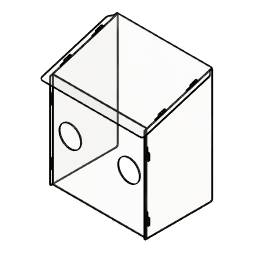
Polycarbinate Box - Flatpack - V5 v38 (Autodesk Fusion 360 design; units mm, degrees)
Autodesk Fusion 360 part; units mm, degrees
note: some values were not read from the file. Set by a fixed rule: which sketch regions a step uses.
ref_plane "WorkPlane1" through (474.6, 0, 0) normal (1, 0, 0) x (0, 1, 0)
ref_plane "WorkPlane2" through (0, 0, 500) normal (0, 0, 1) x (1, 0, 0)
ref_plane "WorkPlane3" through (0, 0, 0) normal (1, 0, 0) x (0, 1, 0)
ref_plane "WorkPlane4" through (0, 400, 0) normal (0, 1, 0) x (0, 0, 1)
sketch "Sketch1" plane through (0, 0, 0) normal (1, 0, 0) x (0, 1, 0)
  line L0 (0, 483.1819) -> (0, 0)
  line L1 (0, 0) -> (390.6577, 0)
  line L2 (9.525, 393.7) -> (14.2875, 393.7)
  line L3 (14.2875, 393.7) -> (14.2875, 355.6)
  line L4 (14.2875, 355.6) -> (9.525, 355.6)
  line L5 (9.525, 355.6) -> (9.525, 393.7)
  line L6 (9.525, 114.3) -> (14.2875, 114.3)
  line L7 (14.2875, 114.3) -> (14.2875, 76.2)
  line L8 (14.2875, 76.2) -> (9.525, 76.2)
  line L9 (9.525, 76.2) -> (9.525, 114.3)
  arc A0 (390.6577, 0) -> (400.1827, 9.525) centre (390.6577, 9.525) ccw
  line L10 (0, 483.1819) -> (336.55, 586.2176)
  line L11 (72.8618, 492.2069) -> (69.144, 504.3505)
  line L12 (104.8626, 506.9847) -> (102.539, 514.5745)
  line L13 (89.5593, 497.3188) -> (88.1651, 501.8727)
  line L14 (104.8626, 506.9847) -> (88.1651, 501.8727)
  line L15 (230.2932, 540.4049) -> (226.5754, 552.5485)
  line L16 (246.9907, 545.5169) -> (245.5965, 550.0707)
  line L17 (245.5965, 550.0707) -> (262.294, 555.1827)
  line L18 (262.294, 555.1827) -> (259.9704, 562.7725)
  line L19 (72.8618, 492.2069) -> (0, 469.9)
  line L20 (336.55, 572.9357) -> (246.9907, 545.5169)
  line L21 (230.2932, 540.4049) -> (89.5593, 497.3188)
  line L22 (336.55, -28.3525) -> (336.55, 572.9357)
  line L23 (89.5593, 497.3188) -> (88.1651, 501.8727)
  dimension "d6" = 9.525
  dimension "d7" = 76.2
  dimension "d8" = 38.1
  dimension "d9" = 4.7625
  dimension "d13" = 9.525
  dimension "d14" = 4.7625
  dimension "d15" = 38.1
  dimension "d31" = 9.525
  dimension "d140" = 76.2
  dimension "d150" = 469.9
  dimension "d151" = 12.7
  dimension "d152" = 76.2
  dimension "d153" = 34.925
  dimension "d154" = 17.4625
  dimension "d155" = 4.7625
  dimension "d160" = 34.925
  dimension "d161" = 17.4625
  dimension "d163" = 4.7625
  dimension "d165" = 76.2
  dimension "d202" = 336.55
  constraint vertical L0
  constraint horizontal L1
  constraint coincident L0.end L1.start
  constraint coincident L0 L19.end
  constraint horizontal L2
  constraint vertical L3
  constraint horizontal L4
  constraint vertical L5
  constraint horizontal L6
  constraint vertical L7
  constraint horizontal L8
  constraint vertical L9
  constraint tangent L1 A0
  constraint perpendicular L1 L22
  constraint coincident L11.start L20
  constraint coincident L10 L11.end
  constraint perpendicular L10 L11
  constraint coincident L10 L12.end
  constraint perpendicular L10 L12
  constraint perpendicular L13 L14
  constraint coincident L10.end L22
  constraint coincident L15.start L20
  constraint coincident L10 L15.end
  constraint perpendicular L10 L15
  constraint perpendicular L16 L20
  constraint perpendicular L16 L17
  constraint coincident L10 L18.end
  constraint perpendicular L10 L18
  constraint collinear L19 L20
  constraint collinear L20 L21
  measures "d6" distance of L0 L9
  measures "d7" distance of L1 L8
  measures "d8" distance of L6.start L8.end
  measures "d9" distance of L7 L9
  measures "d13" distance of L0 L5
  measures "d14" distance of L3 L5
  measures "d15" distance of L2.start L4.end
  measures "d31" radius of A0
  measures "d140" distance of L19.end L2
  measures "d150" distance of L1 L19.end
  measures "d151" distance of L10 L20
  measures "d152" distance of L19.end L11
  measures "d153" distance of L11 L12
  measures "d154" distance of L11 L13
  measures "d155" distance of L14 L20
  measures "d160" distance of L15 L18
  measures "d161" distance of L15 L16
  measures "d163" distance of L17 L20
  measures "d165" distance of L20.start L18
  measures "d202" distance of L0 L22
extrude "Extrude1" add sketch "Sketch1" along normal blind 4.7625 contours L0 L1 L10 L11 L12 L13 L14 L15 L16 L17 L18 L19 L20 L21 L22 L23 makes body 1
fillet "Fillet1" radius 3.175 6 edges at (2.3813, 69.144, 504.3505) (2.3813, 102.539, 514.5745) (2.3813, 104.8626, 506.9847) (2.3813, 226.5754, 552.5485) (2.3813, 259.9704, 562.7725) (2.3813, 262.294, 555.1827) on bodies 1
fillet "Fillet2" radius 1.5875 5 edges at (2.3813, 0, 469.9) (2.3813, 336.55, 572.9357) (2.3813, 0, 0) (2.3813, 72.8618, 492.2069) (2.3813, 230.2932, 540.4049) on bodies 1
fillet "Fillet3" radius 9.525 1 edges at (2.3813, 336.55, 0) on bodies 1
sketch "Sketch2" plane through (4.7625, 0, 0) normal (1, 0, 0) x (0, 1, 0)
  line L0 (1.5875, 0) -> (327.025, 0)
  arc A0 (14.2875, 114.3) -> (11.1125, 114.3) centre (12.7, 114.3) ccw
  line L1 (9.525, 114.3) -> (14.2875, 114.3)
  arc A1 (9.525, 114.3) -> (9.525, 111.125) centre (9.525, 112.7125) ccw
  arc A2 (9.525, 79.375) -> (9.525, 76.2) centre (9.525, 77.7875) ccw
  arc A3 (11.1125, 76.2) -> (14.2875, 76.2) centre (12.7, 76.2) ccw
  arc A4 (9.525, 358.775) -> (9.525, 355.6) centre (9.525, 357.1875) ccw
  line L2 (14.2875, 355.6) -> (9.525, 355.6)
  line L3 (9.525, 355.6) -> (9.525, 393.7)
  line L4 (9.525, 393.7) -> (14.2875, 393.7)
  arc A5 (11.1125, 355.6) -> (14.2875, 355.6) centre (12.7, 355.6) ccw
  arc A6 (14.2875, 393.7) -> (11.1125, 393.7) centre (12.7, 393.7) ccw
  arc A7 (9.525, 393.7) -> (9.525, 390.525) centre (9.525, 392.1125) ccw
  line L5 (14.2875, 393.7) -> (14.2875, 355.6)
  line L6 (336.55, 9.525) -> (336.55, 570.7895)
  arc A8 (327.025, 0) -> (336.55, 9.525) centre (327.025, 9.525) ccw
  arc A9 (336.55, 570.7895) -> (334.4978, 572.3074) centre (334.9625, 570.7895) ccw
  line L7 (334.4978, 572.3074) -> (246.9907, 545.5169)
  line L8 (246.9907, 545.5169) -> (245.5965, 550.0707)
  line L9 (245.5965, 550.0707) -> (259.2581, 554.2533)
  arc A10 (259.2581, 554.2533) -> (261.3645, 558.2186) centre (258.3286, 557.2892) ccw
  line L10 (261.3645, 558.2186) -> (260.8998, 559.7366)
  arc A11 (260.8998, 559.7366) -> (256.9345, 561.843) centre (257.8639, 558.8071) ccw
  line L11 (256.9345, 561.843) -> (229.6113, 553.478)
  arc A12 (229.6113, 553.478) -> (227.5048, 549.5126) centre (230.5407, 550.4421) ccw
  line L12 (227.5048, 549.5126) -> (229.8285, 541.9229)
  arc A13 (228.7752, 539.9402) -> (229.8285, 541.9229) centre (228.3105, 541.4581) ccw
  line L13 (228.7752, 539.9402) -> (89.5593, 497.3188)
  line L14 (89.5593, 497.3188) -> (88.1651, 501.8727)
  line L15 (88.1651, 501.8727) -> (101.8267, 506.0552)
  arc A14 (101.8267, 506.0552) -> (103.9332, 510.0206) centre (100.8973, 509.0911) ccw
  line L16 (103.9332, 510.0206) -> (103.4685, 511.5386)
  arc A15 (103.4685, 511.5386) -> (99.5031, 513.645) centre (100.4326, 510.6091) ccw
  line L17 (99.5031, 513.645) -> (72.1799, 505.2799)
  arc A16 (72.1799, 505.2799) -> (70.0735, 501.3146) centre (73.1094, 502.244) ccw
  line L18 (70.0735, 501.3146) -> (72.3971, 493.7248)
  arc A17 (71.3439, 491.7421) -> (72.3971, 493.7248) centre (70.8791, 493.2601) ccw
  line L19 (71.3439, 491.7421) -> (1.1228, 470.2437)
  arc A18 (1.1228, 470.2437) -> (0, 468.7258) centre (1.5875, 468.7258) ccw
  line L20 (0, 468.7258) -> (0, 1.5875)
  arc A19 (0, 1.5875) -> (1.5875, 0) centre (1.5875, 1.5875) ccw
  arc A20 (248.6324, 551.0002) -> (245.5965, 550.0707) centre (247.1145, 550.5355) ccw
  line L21 (246.0605, 548.5552) -> (242.3336, 547.4142)
  line L22 (246.9899, 545.5193) -> (245.5965, 550.0707)
  arc A21 (246.0605, 548.5552) -> (246.9899, 545.5193) centre (246.5252, 547.0372) ccw
  line L23 (248.6324, 551.0002) -> (247.4641, 554.8162)
  line L24 (14.2875, 355.6) -> (9.525, 355.6)
  line L25 (9.525, 355.6) -> (9.525, 393.7)
  line L26 (9.525, 393.7) -> (14.2875, 393.7)
  line L27 (14.2875, 393.7) -> (14.2875, 355.6)
  line L28 (14.2875, 76.2) -> (9.525, 76.2)
  line L29 (9.525, 76.2) -> (9.525, 114.3)
  line L30 (9.525, 114.3) -> (14.2875, 114.3)
  line L31 (14.2875, 114.3) -> (14.2875, 76.2)
  line L32 (91.201, 502.8022) -> (90.0328, 506.6182)
  arc A22 (88.6291, 500.3571) -> (89.5586, 497.3212) centre (89.0939, 498.8392) ccw
  arc A23 (91.201, 502.8022) -> (88.1651, 501.8727) centre (89.6831, 502.3374) ccw
  line L33 (88.6291, 500.3571) -> (84.9022, 499.2161)
  dimension "d173" = 3.175
  constraint coincident L21.start L22
  constraint perpendicular L21 L22
  constraint tangent A20 L23
  constraint tangent A20 L22
  constraint tangent L21 A21
  constraint coincident L22.start A21.end
  constraint tangent L32 A23
  constraint tangent A22 L33
  measures "d173" distance of L22 L23
extrude "Extrude2" cut sketch "Sketch2" against normal blind 7.62 contours L8 L22 A21 | L9 A20 | L15 A23 | L14 A22 | A0 L1 L30 | A3 L28 | A1 L29 | A2 L29 | A4 L3 L25 | L3 A7 L25 | L2 A5 L24 | L4 A6 L26 bodies 1
ref_plane "WorkPlane5" through (237.3, 168.275, 286.4678) normal (-1, 0, 0) x (0, -1, 0)
mirror "Mirror1" about plane through (237.3, 168.275, 286.4678) normal (-1, 0, 0) of bodies 1 makes body 2
sketch "Sketch3" plane through (0, 14.2875, 0) normal (0, -1, 0) x (1, 0, 0)
  line L0 (495.2375, 0) -> (4.7625, 0)
  line L1 (4.7625, 474.2742) -> (469.8375, 474.2742)
  line L2 (237.3, 644.4156) -> (237.3, -18.4393)
  line L3 (4.7625, 76.2) -> (4.7625, 0)
  line L4 (4.7625, 1.5875) -> (4.7625, 0)
  line L5 (4.7625, 9.525) -> (4.7625, 0)
  line L6 (4.7625, 93.6625) -> (-9.525, 93.6625)
  line L7 (-9.525, 93.6625) -> (-9.525, 58.7375)
  line L8 (-9.525, 58.7375) -> (0, 58.7375)
  line L9 (0, 58.7375) -> (0, 76.2)
  line L10 (0, 76.2) -> (4.7625, 76.2)
  line L11 (0, 393.7) -> (0, 355.6)
  line L12 (0, 355.6) -> (4.7625, 355.6)
  line L13 (4.7625, 355.6) -> (4.7625, 393.7)
  line L14 (4.7625, 393.7) -> (0, 393.7)
  line L15 (-9.525, 373.0625) -> (-9.525, 338.1375)
  line L16 (0, 355.6) -> (4.7625, 355.6)
  line L17 (4.7625, 373.0625) -> (0, 373.0625)
  line L18 (4.7625, 373.0625) -> (-9.525, 373.0625)
  line L19 (0, 338.1375) -> (0, 355.6)
  line L20 (-9.525, 338.1375) -> (0, 338.1375)
  line L21 (4.7625, 373.0625) -> (4.7625, 474.2742)
  line L22 (4.7625, 355.6) -> (4.7625, 93.6625)
  line L23 (0, 114.3) -> (0, 76.2)
  line L24 (0, 76.2) -> (4.7625, 76.2)
  line L25 (4.7625, 76.2) -> (4.7625, 114.3)
  line L26 (4.7625, 114.3) -> (0, 114.3)
  line L27 (237.3, 474.2742) -> (237.3, 298.45)
  line L28 (4.7625, 474.2742) -> (0, 474.2742)
  line L29 (4.7625, 500.3571) -> (4.7625, 501.8727)
  line L30 (469.8375, 497.3212) -> (469.8375, 497.3188)
  line L31 (469.8375, 545.5193) -> (469.8375, 545.5169)
  line L32 (474.6, 393.7) -> (474.6, 355.6)
  line L33 (474.6, 76.2) -> (469.8375, 76.2)
  line L34 (474.6, 355.6) -> (469.8375, 355.6)
  line L35 (474.6, 114.3) -> (474.6, 76.2)
  line L36 (474.6, 355.6) -> (469.8375, 355.6)
  line L37 (474.6, 338.1375) -> (474.6, 355.6)
  line L38 (469.8375, 373.0625) -> (469.8375, 474.2742)
  line L39 (469.8375, 474.2742) -> (474.6, 474.2742)
  line L40 (484.125, 373.0625) -> (484.125, 338.1375)
  line L41 (469.8375, 76.2) -> (469.8375, 114.3)
  line L42 (469.8375, 355.6) -> (469.8375, 93.6625)
  line L43 (484.125, 338.1375) -> (474.6, 338.1375)
  line L44 (469.8375, 373.0625) -> (474.6, 373.0625)
  line L45 (469.8375, 76.2) -> (469.8375, 0)
  line L46 (484.125, 58.7375) -> (474.6, 58.7375)
  line L47 (469.8375, 373.0625) -> (484.125, 373.0625)
  line L48 (469.8375, 1.5875) -> (469.8375, 0)
  line L49 (469.8375, 393.7) -> (474.6, 393.7)
  line L50 (474.6, 58.7375) -> (474.6, 76.2)
  line L51 (469.8375, 500.3571) -> (469.8375, 501.8727)
  line L52 (469.8375, 93.6625) -> (484.125, 93.6625)
  line L53 (484.125, 93.6625) -> (484.125, 58.7375)
  line L54 (469.8375, 114.3) -> (474.6, 114.3)
  line L55 (469.8375, 9.525) -> (469.8375, 0)
  line L56 (474.6, 76.2) -> (469.8375, 76.2)
  line L57 (469.8375, 355.6) -> (469.8375, 393.7)
  line L58 (4.7625, 548.5552) -> (4.7625, 550.0707)
  arc A0 (4.7625, 355.6) -> (1.5875, 355.6) centre (3.175, 355.6) ccw
  arc A1 (0, 355.6) -> (0, 352.425) centre (0, 354.0125) ccw
  arc A2 (4.7625, 76.2) -> (1.5875, 76.2) centre (3.175, 76.2) ccw
  arc A3 (0, 76.2) -> (0, 73.025) centre (0, 74.6125) ccw
  arc A4 (473.0125, 76.2) -> (469.8375, 76.2) centre (471.425, 76.2) ccw
  arc A5 (474.6, 73.025) -> (474.6, 76.2) centre (474.6, 74.6125) ccw
  arc A6 (473.0125, 355.6) -> (469.8375, 355.6) centre (471.425, 355.6) ccw
  arc A7 (474.6, 352.425) -> (474.6, 355.6) centre (474.6, 354.0125) ccw
  point P0 (4.7625, 393.7)
  point P1 (4.7625, 355.6)
  point P2 (4.7625, 114.3)
  point P3 (4.7625, 76.2)
  point P4 (469.8375, 355.6)
  point P5 (469.8375, 76.2)
  point P6 (469.8375, 0)
  point P7 (469.8375, 114.3)
  point P8 (474.6, 0)
  point P9 (469.8375, 393.7)
  dimension "d203" = 34.925
  dimension "d204" = 17.4625
  dimension "d206" = 34.925
  dimension "d207" = 17.4625
  dimension "d226" = 232.5375
  dimension "d227" = 232.5375
  dimension "d228" = 3.175
  dimension "d229" = 3.175
  dimension "d230" = 3.175
  dimension "d231" = 3.175
  dimension "d232" = 3.175
  dimension "d234" = 1.5875
  dimension "d235" = 1.5875
  dimension "d236" = 1.5875
  constraint coincident L0.end L3.end
  constraint perpendicular L6 L7
  constraint perpendicular L15 L18
  constraint perpendicular L1 L21
  constraint midpoint L1 L27.start
  constraint coincident L2 L27.end
  constraint perpendicular L1 L27
  constraint symmetric origin L2 P8
  constraint symmetric L0.end L2 P6
  constraint symmetric L1.start L2 L1.end
  constraint symmetric L2 L0.end P6
  constraint symmetric L2 L4.start L48.start
  constraint symmetric L2 L5.start L55.start
  constraint symmetric L2 L6.start L42.end
  constraint symmetric L2 L6.end L52.end
  constraint symmetric L2 L7.end L46.start
  constraint symmetric L2 L8.end L46.end
  constraint symmetric L2 L9.end L33.start
  constraint symmetric L2 P3 P5
  constraint symmetric L2 L11.start L32.start
  constraint symmetric L2 L11.end L32.end
  constraint symmetric L2 P1 P4
  constraint symmetric L2 P0 P9
  constraint symmetric L2 L17.end L44.end
  constraint symmetric L2 L17.start L38.start
  constraint symmetric L2 L15.start L40.start
  constraint symmetric L2 L19.start L37.start
  constraint symmetric L2 L15.end L40.end
  constraint symmetric L2 L23.start L35.start
  constraint symmetric L2 P2 P7
  constraint symmetric L2 L1.start L1.end
  constraint symmetric L2 L28.end L39.end
  constraint symmetric L2 L29.start L51.start
  constraint symmetric L2 L29.end L51.end
  constraint tangent L13 A0
  constraint coincident L12 A0.end
  constraint coincident P1 L12.end
  constraint tangent L16 A1
  constraint coincident L19 A1.end
  constraint coincident L11.end L12.start
  constraint tangent L3 A2
  constraint tangent L25 A2
  constraint coincident L24 A2.end
  constraint coincident P3 L3.start
  constraint tangent L24 A3
  constraint coincident L9 A3.end
  constraint coincident L9.end L10.start
  constraint tangent L41 A4
  constraint coincident L56 A4.start
  constraint tangent L33 A5
  constraint coincident L50 A5.start
  constraint tangent L57 A6
  constraint coincident L34 A6.start
  constraint tangent L34 A7
  constraint coincident L37 A7.start
  measures "d203" distance of L6.end L7.end
  measures "d204" distance of L8 L10
  measures "d206" distance of L15.start L15.end
  measures "d207" distance of L16 L20
  measures "d226" distance of L2 L22
  measures "d227" distance of L27 L38
  measures "d228" distance of L16 A1.end
  measures "d229" distance of L22 A0.end
  measures "d230" distance of L3 A2.end
  measures "d231" distance of L10 A3.end
  measures "d232" distance of L45 A4.start
  measures "d234" radius of A5
  measures "d235" radius of A6
  measures "d236" radius of A7
extrude "Extrude3" add sketch "Sketch3" along normal blind 4.7752 separate body contours L0 L1 L2 L27 L38 L41 L42 L45 L48 L55 L57 | L0 L1 L2 L3 L4 L5 L13 L21 L22 L25 L27 | L33 L35 L41 L52 L56 A4 | L6 L10 L23 L24 L25 A2 | L35 L46 L50 L52 L53 A5 | L11 L12 L13 L16 L17 L18 A0 | L32 L34 L36 L44 L47 L57 A6 | L6 L7 L8 L9 L23 A3 | L11 L15 L18 L19 L20 A1 | L32 L37 L40 L43 L47 A7 makes body 3
fillet "Fillet5" radius 3.175 12 edges at (-9.525, 11.8999, 373.0625) (-9.525, 11.8999, 338.1375) (0, 11.8999, 338.1375) (-9.525, 11.8999, 93.6625) (-9.525, 11.8999, 58.7375) (0, 11.8999, 58.7375) (474.6, 11.8999, 338.1375) (484.125, 11.8999, 338.1375) (484.125, 11.8999, 373.0625) (484.125, 11.8999, 93.6625) (484.125, 11.8999, 58.7375) (474.6, 11.8999, 58.7375) on bodies 3
fillet "Fillet6" radius 1.5875 4 edges at (4.7625, 11.8999, 93.6625) (4.7625, 11.8999, 373.0625) (469.8375, 11.8999, 93.6625) (469.8375, 11.8999, 373.0625) on bodies 3
sketch "Sketch5" plane through (0, -131.5327, 429.6309) normal (0, -0.292741, 0.956192) x (1, 0, 0)
  line L0 (0, 213.7589) -> (4.7625, 213.7589)
  line L1 (4.7625, 213.7589) -> (0, 213.7589)
  line L2 (4.7625, 376.8155) -> (0, 376.8155)
  line L3 (0, 376.8155) -> (0, 231.2214)
  line L4 (4.7625, 231.2214) -> (4.7625, 376.8155)
  line L5 (0, 378.403) -> (4.7625, 378.403)
  line L6 (4.7625, 378.403) -> (0, 378.403)
  line L7 (4.7625, 487.3817) -> (0, 487.3817)
  line L8 (0, 487.3817) -> (0, 395.8655)
  line L9 (4.7625, 395.8655) -> (4.7625, 487.3817)
  line L10 (474.6, 487.3817) -> (469.8375, 487.3817)
  line L11 (469.8375, 487.3817) -> (469.8375, 395.8655)
  line L12 (474.6, 395.8655) -> (474.6, 487.3817)
  line L13 (469.8375, 378.403) -> (474.6, 378.403)
  line L14 (474.6, 378.403) -> (469.8375, 378.403)
  line L15 (474.6, 376.8155) -> (469.8375, 376.8155)
  line L16 (469.8375, 376.8155) -> (469.8375, 231.2214)
  line L17 (474.6, 231.2214) -> (474.6, 376.8155)
  line L18 (469.8375, 213.7589) -> (474.6, 213.7589)
  line L19 (474.6, 213.7589) -> (469.8375, 213.7589)
  line L20 (474.6, 212.1714) -> (469.8375, 212.1714)
  line L21 (469.8375, 212.1714) -> (469.8375, 138.7331)
  line L22 (474.6, 138.7331) -> (474.6, 212.1714)
  line L23 (469.8375, 231.2214) -> (474.6, 231.2214)
  line L24 (474.6, 231.2214) -> (474.6, 193.1214)
  line L25 (474.6, 193.1214) -> (469.8375, 193.1214)
  line L26 (469.8375, 193.1214) -> (469.8375, 231.2214)
  line L27 (469.8375, 395.8655) -> (474.6, 395.8655)
  line L28 (474.6, 395.8655) -> (474.6, 357.7655)
  line L29 (474.6, 357.7655) -> (469.8375, 357.7655)
  line L30 (469.8375, 357.7655) -> (469.8375, 395.8655)
  line L31 (0, 395.8655) -> (4.7625, 395.8655)
  line L32 (4.7625, 395.8655) -> (4.7625, 357.7655)
  line L33 (4.7625, 357.7655) -> (0, 357.7655)
  line L34 (0, 357.7655) -> (0, 395.8655)
  line L35 (4.7625, 212.1714) -> (4.7625, 138.7331)
  line L36 (0, 231.2214) -> (4.7625, 231.2214)
  line L37 (4.7625, 231.2214) -> (4.7625, 193.1214)
  line L38 (4.7625, 193.1214) -> (0, 193.1214)
  line L39 (0, 193.1214) -> (0, 231.2214)
  line L40 (493.65, 106.4136) -> (493.65, 457.9634)
  line L41 (493.65, 457.9634) -> (-19.05, 457.9634)
  line L42 (-19.05, 106.4136) -> (-19.05, 457.9634)
  line L43 (-19.05, 106.4136) -> (493.65, 106.4136)
  line L44 (474.6, 324.5947) -> (469.8375, 324.5947)
  line L45 (469.8375, 324.5947) -> (469.8375, 488.8997)
  line L46 (469.8375, 488.8997) -> (474.6, 488.8997)
  line L47 (474.6, 488.8997) -> (474.6, 324.5947)
  line L48 (4.7625, 324.5947) -> (0, 324.5947)
  line L49 (0, 324.5947) -> (0, 488.8997)
  line L50 (0, 488.8997) -> (4.7625, 488.8997)
  line L51 (4.7625, 488.8997) -> (4.7625, 324.5947)
  line L52 (474.6, 488.8997) -> (493.65, 488.8997)
  line L53 (469.8375, 488.8997) -> (4.7625, 488.8997)
  line L54 (0, 488.8997) -> (-19.05, 488.8997)
  line L55 (0, 488.8997) -> (0, 457.9634)
  line L56 (237.3, 457.9634) -> (237.3, 482.6)
  line L57 (474.6, 488.8997) -> (474.6, 457.9634)
  line L58 (0, 476.1997) -> (-19.05, 457.1497)
  line L59 (474.6, 476.1997) -> (493.65, 457.1497)
  line L60 (0, 231.2214) -> (4.7625, 231.2214)
  line L61 (0, 395.8655) -> (4.7625, 395.8655)
  line L62 (469.8375, 395.8655) -> (474.6, 395.8655)
  line L63 (469.8375, 231.2214) -> (474.6, 231.2214)
  line L64 (4.7625, 147.507) -> (469.8375, 147.507)
  point P0 (0, 213.7589)
  point P1 (0, 378.403)
  point P2 (469.8375, 378.403)
  point P3 (469.8375, 213.7589)
  dimension "d210" = 38.1
  dimension "d211" = 38.1
  dimension "d212" = 38.1
  dimension "d213" = 38.1
  dimension "d214" = 19.05
  dimension "d215" = 19.05
  dimension "d222" = 12.7
  dimension "d223" = 45
  constraint horizontal L23
  constraint vertical L24
  constraint horizontal L25
  constraint vertical L26
  constraint coincident L22 L24.end
  constraint coincident L16.end L23.start
  constraint horizontal L27
  constraint vertical L28
  constraint horizontal L29
  constraint vertical L30
  constraint coincident L17 L28.end
  constraint coincident L11.end L27.start
  constraint horizontal L31
  constraint vertical L32
  constraint horizontal L33
  constraint vertical L34
  constraint coincident L4 L32.end
  constraint coincident L8.end L31.start
  constraint horizontal L36
  constraint vertical L37
  constraint horizontal L38
  constraint vertical L39
  constraint coincident L35 L37.end
  constraint coincident L3.end L36.start
  constraint perpendicular L22 L41
  constraint perpendicular L42 L43
  constraint coincident L46.end L47.start
  constraint coincident L40 L52.end
  constraint perpendicular L40 L52
  constraint coincident L45.end L46.start
  constraint coincident L50.end L51.start
  constraint coincident L49.end L50.start
  constraint coincident L42 L54.end
  constraint perpendicular L42 L54
  constraint coincident L41 L55.end
  constraint perpendicular L41 L55
  constraint midpoint L41 L56.start
  constraint perpendicular L41 L56
  constraint symmetric L49.end L56 L46.end
  constraint coincident L41 L57.end
  constraint perpendicular L41 L57
  constraint coincident L8 L58.start
  constraint coincident L42 L58.end
  constraint symmetric L56 L58.start L59.start
  constraint symmetric L56 L58.end L59.end
  measures "d210" distance of L16.end L25.end
  measures "d211" distance of L11.end L29.end
  measures "d212" distance of L8.end L33.end
  measures "d213" distance of L3.end L38.end
  measures "d214" distance of L8 L42
  measures "d215" distance of L12 L40
  measures "d222" distance of L49.end L58.start
  measures "d223" angle of L49 L58
extrude "Extrude5" add sketch "Sketch5" along normal blind 4.7625 separate body contours L3 L8 L12 L17 L21 L22 L24 L25 L28 L34 L35 L38 L39 L40 L41 L42 L43 L47 L49 L58 L59 L64 | L4 L9 L11 L16 L21 L26 L30 L32 L35 L37 L41 L45 L51 L64 | L3 L4 L36 L48 L60 | L3 L4 L33 L48 L49 L51 | L8 L9 L31 L41 L49 L51 L61 | L8 L41 L49 L55 L58 | L7 L8 L9 L41 L49 L51 L55 | L9 L11 L41 L45 L51 L53 | L16 L17 L23 L44 L63 | L7 L49 L50 L51 L55 | L16 L17 L29 L44 L45 L47 | L11 L12 L27 L41 L45 L47 L62 | L10 L11 L12 L41 L45 L47 L57 | L10 L45 L46 L47 L57 | L12 L41 L47 L57 L59 makes body 4
fillet "Fillet7" radius 12.7 6 edges at (493.65, -30.478, 463.0594) (-19.05, -30.478, 463.0594) (474.6, 323.1085, 571.3109) (493.65, 304.8931, 565.7341) (0, 323.1085, 571.3109) (-19.05, 304.8931, 565.7341) on bodies 4
fillet "Fillet15" radius 1.5875 2 edges at (0, 335.2522, 575.0287) (474.6, 335.2522, 575.0287) on bodies 4
sketch "Sketch6" plane through (0, 9.5123, 0) normal (0, -1, 0) x (1, 0, 0)
  line L0 (4.7625, 76.2) -> (4.7625, 0)
  line L1 (4.7625, 0) -> (469.8375, 0)
  line L2 (-14.0434, 355.9906) -> (-14.1038, 359.0206)
  line L3 (-14.4856, 352.0297) -> (-16.2729, 352.0041)
  arc A0 (-9.102, 355.8831) -> (-14.0434, 355.9906) centre (-11.5704, 356.04) ccw
  arc A1 (-13.3885, 355.7513) -> (-14.4856, 352.0297) centre (-14.5148, 354.0608) ccw
  line L4 (-12.7077, 76.6564) -> (-7.945, 76.6928)
  arc A2 (-7.7782, 76.2457) -> (-12.8158, 76.6555) centre (-10.2787, 76.6749) ccw
  arc A3 (-12.6794, 76.6556) -> (-12.5673, 70.6711) centre (-12.7327, 73.6613) ccw
  line L5 (-12.8158, 76.6555) -> (-12.838, 79.5692)
  line L6 (237.3, 0) -> (237.3, 64.7378)
  line L7 (4.7625, 474.2742) -> (4.7625, 374.65)
  arc A4 (3.175, 373.0625) -> (4.7625, 374.65) centre (3.175, 374.65) ccw
  line L8 (3.175, 373.0625) -> (-6.35, 373.0625)
  arc A5 (-6.35, 373.0625) -> (-9.525, 369.8875) centre (-6.35, 369.8875) ccw
  line L9 (-9.525, 369.8875) -> (-9.525, 341.3125)
  arc A6 (-9.525, 341.3125) -> (-6.35, 338.1375) centre (-6.35, 341.3125) ccw
  line L10 (-6.35, 338.1375) -> (-3.175, 338.1375)
  arc A7 (-3.175, 338.1375) -> (0, 341.3125) centre (-3.175, 341.3125) ccw
  line L11 (0, 341.3125) -> (0, 352.425)
  line L12 (0, 355.6) -> (1.5875, 355.6)
  line L13 (4.7625, 355.6) -> (4.7625, 114.3)
  arc A8 (3.175, 93.6625) -> (4.7625, 95.25) centre (3.175, 95.25) ccw
  line L14 (3.175, 93.6625) -> (-6.35, 93.6625)
  arc A9 (-6.35, 93.6625) -> (-9.525, 90.4875) centre (-6.35, 90.4875) ccw
  line L15 (-9.525, 90.4875) -> (-9.525, 61.9125)
  arc A10 (-9.525, 61.9125) -> (-6.35, 58.7375) centre (-6.35, 61.9125) ccw
  line L16 (-6.35, 58.7375) -> (-3.175, 58.7375)
  arc A11 (-3.175, 58.7375) -> (0, 61.9125) centre (-3.175, 61.9125) ccw
  line L17 (0, 61.9125) -> (0, 73.025)
  line L18 (0, 76.2) -> (1.5875, 76.2)
  line L19 (4.7625, 114.3) -> (4.7625, 95.25)
  line L20 (469.8375, 393.7) -> (469.8375, 474.2742)
  arc A12 (0, 355.6) -> (0, 352.425) centre (0, 354.0125) ccw
  arc A13 (4.7625, 355.6) -> (1.5875, 355.6) centre (3.175, 355.6) ccw
  arc A14 (0, 76.2) -> (0, 73.025) centre (0, 74.6125) ccw
  arc A15 (4.7625, 76.2) -> (1.5875, 76.2) centre (3.175, 76.2) ccw
  arc A16 (473.0125, 76.2) -> (469.8375, 76.2) centre (471.425, 76.2) ccw
  arc A17 (474.6, 73.025) -> (474.6, 76.2) centre (474.6, 74.6125) ccw
  arc A18 (473.0125, 355.6) -> (469.8375, 355.6) centre (471.425, 355.6) ccw
  arc A19 (474.6, 352.425) -> (474.6, 355.6) centre (474.6, 354.0125) ccw
  line L21 (469.8375, 474.2742) -> (4.7625, 474.2742)
  constraint tangent L2 A0
  constraint tangent L3 A1
  constraint coincident A2.end L4
  constraint perpendicular L4 L5
  constraint tangent A2 L5
  constraint tangent L4 A3
  constraint midpoint L1 L6.start
  constraint perpendicular L1 L6
extrude "Extrude6" cut sketch "Sketch6" against normal blind 6.35 bodies 3
sketch "Sketch7" plane through (0, -132.9268, 434.1848) normal (0, -0.292741, 0.956192) x (1, 0, 0)
  arc A0 (4.7625, 372.7971) -> (1.5875, 372.7971) centre (3.175, 372.7971) ccw
  arc A1 (0, 372.7971) -> (0, 369.6221) centre (0, 371.2096) ccw
  arc A2 (1.5875, 334.6971) -> (4.7625, 334.6971) centre (3.175, 334.6971) ccw
  arc A3 (0, 337.8721) -> (0, 334.6971) centre (0, 336.2846) ccw
  line L0 (250, 501.1312) -> (250, 406.4)
  arc A4 (4.7625, 183.778) -> (1.5875, 183.778) centre (3.175, 183.778) ccw
  arc A5 (0, 183.778) -> (0, 180.603) centre (0, 182.1905) ccw
  arc A6 (0, 148.853) -> (0, 145.678) centre (0, 147.2655) ccw
  arc A7 (1.5875, 145.678) -> (4.7625, 145.678) centre (3.175, 145.678) ccw
  line L1 (0, 357.7655) -> (0, 395.8655)
  line L2 (4.7625, 395.8655) -> (4.7625, 357.7655)
  line L3 (4.7625, 193.1214) -> (0, 193.1214)
  line L4 (0, 193.1214) -> (0, 231.2214)
  line L5 (0, 231.2214) -> (4.7625, 231.2214)
  line L6 (4.7625, 231.2214) -> (4.7625, 193.1214)
  line L7 (-19.05, 451.8892) -> (-19.05, 119.1136)
  arc A8 (500, 145.678) -> (500, 148.853) centre (500, 147.2655) ccw
  arc A9 (500, 369.6221) -> (500, 372.7971) centre (500, 371.2096) ccw
  line L8 (500, 193.1214) -> (500, 231.2214)
  line L9 (495.2375, 193.1214) -> (500, 193.1214)
  line L10 (495.2375, 231.2214) -> (495.2375, 193.1214)
  arc A10 (498.4125, 372.7971) -> (495.2375, 372.7971) centre (496.825, 372.7971) ccw
  arc A11 (495.2375, 145.678) -> (498.4125, 145.678) centre (496.825, 145.678) ccw
  arc A12 (500, 180.603) -> (500, 183.778) centre (500, 182.1905) ccw
  line L11 (495.2375, 357.7655) -> (500, 357.7655)
  arc A13 (498.4125, 183.778) -> (495.2375, 183.778) centre (496.825, 183.778) ccw
  line L12 (500, 357.7655) -> (500, 395.8655)
  line L13 (500, 231.2214) -> (495.2375, 231.2214)
  line L14 (500, 395.8655) -> (495.2375, 395.8655)
  arc A14 (495.2375, 334.6971) -> (498.4125, 334.6971) centre (496.825, 334.6971) ccw
  line L15 (495.2375, 395.8655) -> (495.2375, 357.7655)
  arc A15 (500, 334.6971) -> (500, 337.8721) centre (500, 336.2846) ccw
  line L16 (-6.35, 106.4136) -> (480.95, 106.4136)
  arc A16 (-19.05, 119.1136) -> (-6.35, 106.4136) centre (-6.35, 119.1136) ccw
  arc A17 (480.95, 106.4136) -> (493.65, 119.1136) centre (480.95, 119.1136) ccw
  line L17 (473.0125, 488.8997) -> (1.5875, 488.8997)
  line L18 (489.9303, 460.8694) -> (478.3197, 472.4799)
  line L19 (474.6, 481.4602) -> (474.6, 487.3122)
  line L20 (0, 487.3122) -> (0, 481.4602)
  line L21 (-3.7197, 472.4799) -> (-15.3303, 460.8694)
  line L22 (0, 395.8655) -> (4.7625, 395.8655)
  arc A18 (-15.3303, 460.8694) -> (-19.05, 451.8892) centre (-6.35, 451.8892) ccw
  arc A19 (493.65, 451.8892) -> (489.9303, 460.8694) centre (480.95, 451.8892) ccw
  arc A20 (474.6, 481.4602) -> (478.3197, 472.4799) centre (487.3, 481.4602) ccw
  arc A21 (-3.7197, 472.4799) -> (0, 481.4602) centre (-12.7, 481.4602) ccw
  arc A22 (474.6, 487.3122) -> (473.0125, 488.8997) centre (473.0125, 487.3122) ccw
  arc A23 (1.5875, 488.8997) -> (0, 487.3122) centre (1.5875, 487.3122) ccw
  line L23 (4.7625, 357.7655) -> (0, 357.7655)
  constraint symmetric A0.end L0 A10.start
  constraint symmetric A1.end L0 A9.start
  constraint symmetric A0.start L0 A10.end
  constraint symmetric A0 L0 A10
  constraint symmetric A1.start L0 A9.end
  constraint symmetric A1 L0 A9
  constraint symmetric A2.end L0 A14.start
  constraint symmetric A2.start L0 A14.end
  constraint symmetric A2 L0 A14
  constraint symmetric A3.end L0 A15.start
  constraint symmetric A3.start L0 A15.end
  constraint symmetric A3 L0 A15
  constraint symmetric L0 A4.start A13.end
  constraint symmetric L0 A5.start A12.end
  constraint symmetric L0 A5.end A12.start
  constraint symmetric L0 A6.start A8.end
  constraint symmetric L0 A4.end A13.start
  constraint symmetric L0 A7.end A11.start
  constraint symmetric L0 A7.start A11.end
  constraint symmetric L0 A6.end A8.start
  constraint symmetric L0 A4 A13
  constraint symmetric L0 A5 A12
  constraint symmetric L0 A6 A8
  constraint symmetric L0 A7 A11
  constraint symmetric L0 L2.end L11.start
  constraint symmetric L0 L1.start L11.end
  constraint symmetric L0 L1.end L12.end
  constraint symmetric L0 L2.start L14.end
  constraint symmetric L0 L3.start L9.start
  constraint symmetric L0 L3.end L8.start
  constraint symmetric L0 L4.end L8.end
  constraint symmetric L0 L5.end L10.start
extrude "Extrude7" cut sketch "Sketch7" against normal blind 11.43 contours A1 L1 | A9 L12 bodies 4
sketch "Sketch8" plane through (0, 9.5123, 0) normal (0, -1, 0) x (1, 0, 0)
  line L0 (4.7625, 76.2) -> (4.7625, 0)
  line L1 (4.7625, 0) -> (469.8375, 0)
  circle A0 centre (91.1225, 250) radius 53.975
  circle A1 centre (383.4775, 250) radius 53.975
  line L2 (4.7625, 474.2742) -> (4.7625, 374.65)
  arc A2 (3.175, 373.0625) -> (4.7625, 374.65) centre (3.175, 374.65) ccw
  line L3 (3.175, 373.0625) -> (-6.35, 373.0625)
  arc A3 (-6.35, 373.0625) -> (-9.525, 369.8875) centre (-6.35, 369.8875) ccw
  line L4 (-9.525, 369.8875) -> (-9.525, 341.3125)
  arc A4 (-9.525, 341.3125) -> (-6.35, 338.1375) centre (-6.35, 341.3125) ccw
  line L5 (-6.35, 338.1375) -> (-3.175, 338.1375)
  arc A5 (-3.175, 338.1375) -> (0, 341.3125) centre (-3.175, 341.3125) ccw
  line L6 (0, 341.3125) -> (0, 352.425)
  line L7 (0, 355.6) -> (1.5875, 355.6)
  line L8 (4.7625, 355.6) -> (4.7625, 114.3)
  arc A6 (3.175, 93.6625) -> (4.7625, 95.25) centre (3.175, 95.25) ccw
  line L9 (3.175, 93.6625) -> (-6.35, 93.6625)
  arc A7 (-6.35, 93.6625) -> (-9.525, 90.4875) centre (-6.35, 90.4875) ccw
  line L10 (-9.525, 90.4875) -> (-9.525, 61.9125)
  arc A8 (-9.525, 61.9125) -> (-6.35, 58.7375) centre (-6.35, 61.9125) ccw
  line L11 (-6.35, 58.7375) -> (-3.175, 58.7375)
  arc A9 (-3.175, 58.7375) -> (0, 61.9125) centre (-3.175, 61.9125) ccw
  line L12 (0, 61.9125) -> (0, 73.025)
  line L13 (0, 76.2) -> (1.5875, 76.2)
  line L14 (473.0125, 76.2) -> (474.6, 76.2)
  line L15 (474.6, 73.025) -> (474.6, 61.9125)
  arc A10 (474.6, 61.9125) -> (477.775, 58.7375) centre (477.775, 61.9125) ccw
  line L16 (477.775, 58.7375) -> (480.95, 58.7375)
  arc A11 (480.95, 58.7375) -> (484.125, 61.9125) centre (480.95, 61.9125) ccw
  line L17 (484.125, 61.9125) -> (484.125, 90.4875)
  arc A12 (484.125, 90.4875) -> (480.95, 93.6625) centre (480.95, 90.4875) ccw
  line L18 (480.95, 93.6625) -> (471.425, 93.6625)
  arc A13 (469.8375, 95.25) -> (471.425, 93.6625) centre (471.425, 95.25) ccw
  line L19 (469.8375, 95.25) -> (469.8375, 355.6)
  line L20 (473.0125, 355.6) -> (474.6, 355.6)
  line L21 (474.6, 352.425) -> (474.6, 341.3125)
  arc A14 (474.6, 341.3125) -> (477.775, 338.1375) centre (477.775, 341.3125) ccw
  line L22 (477.775, 338.1375) -> (480.95, 338.1375)
  arc A15 (480.95, 338.1375) -> (484.125, 341.3125) centre (480.95, 341.3125) ccw
  line L23 (484.125, 341.3125) -> (484.125, 369.8875)
  arc A16 (484.125, 369.8875) -> (480.95, 373.0625) centre (480.95, 369.8875) ccw
  line L24 (480.95, 373.0625) -> (471.425, 373.0625)
  arc A17 (469.8375, 374.65) -> (471.425, 373.0625) centre (471.425, 374.65) ccw
  line L25 (469.8375, 374.65) -> (469.8375, 393.7)
  line L26 (469.8375, 0) -> (469.8375, 76.2)
  line L27 (4.7625, 114.3) -> (4.7625, 95.25)
  line L28 (469.8375, 393.7) -> (469.8375, 474.2742)
  arc A18 (0, 355.6) -> (0, 352.425) centre (0, 354.0125) ccw
  arc A19 (4.7625, 355.6) -> (1.5875, 355.6) centre (3.175, 355.6) ccw
  arc A20 (0, 76.2) -> (0, 73.025) centre (0, 74.6125) ccw
  arc A21 (4.7625, 76.2) -> (1.5875, 76.2) centre (3.175, 76.2) ccw
  arc A22 (473.0125, 76.2) -> (469.8375, 76.2) centre (471.425, 76.2) ccw
  arc A23 (474.6, 73.025) -> (474.6, 76.2) centre (474.6, 74.6125) ccw
  arc A24 (473.0125, 355.6) -> (469.8375, 355.6) centre (471.425, 355.6) ccw
  arc A25 (474.6, 352.425) -> (474.6, 355.6) centre (474.6, 354.0125) ccw
  line L29 (469.8375, 474.2742) -> (4.7625, 474.2742)
  dimension "d92" = 250
  dimension "d93" = 107.95
  dimension "d94" = 107.95
  dimension "d97" = 250
  dimension "d218" = 86.36
  dimension "d225" = 86.36
  measures "d92" distance of L1 A0.centre
  measures "d93" diameter of A0
  measures "d94" diameter of A1
  measures "d97" distance of L1 A1.centre
  measures "d218" distance of A0.centre L8
  measures "d225" distance of A1.centre L19
extrude "Extrude8" cut sketch "Sketch8" against normal blind 38.1 contours A0 | A1 bodies 3
copy_body "Body->Comp1" bodies 1 removing the originals makes body 5 in component "Left Side"
copy_body "Body->Comp2" bodies 2 removing the originals makes body 6 in component "Right Side"
copy_body "Body->Comp3" bodies 3 removing the originals makes body 7 in component "Front"
copy_body "Body->Comp4" bodies 4 removing the originals makes body 8 in component "Top"
sketch "Front" plane through (0, 9.5123, 0) normal (0, -1, 0) x (1, 0, 0)
  circle A0 centre (408.8775, 250) radius 53.975
  circle A1 centre (91.1225, 250) radius 53.975
  arc A2 (498.4125, 76.2) -> (495.2375, 76.2) centre (496.825, 76.2) ccw
  arc A3 (500, 73.025) -> (500, 76.2) centre (500, 74.6125) ccw
  arc A4 (498.4125, 355.6) -> (495.2375, 355.6) centre (496.825, 355.6) ccw
  arc A5 (500, 352.425) -> (500, 355.6) centre (500, 354.0125) ccw
  line L0 (4.7625, 472.8122) -> (4.7625, 374.65)
  arc A6 (3.175, 373.0625) -> (4.7625, 374.65) centre (3.175, 374.65) ccw
  line L1 (3.175, 373.0625) -> (-6.35, 373.0625)
  arc A7 (-6.35, 373.0625) -> (-9.525, 369.8875) centre (-6.35, 369.8875) ccw
  line L2 (-9.525, 369.8875) -> (-9.525, 341.3125)
  arc A8 (-9.525, 341.3125) -> (-6.35, 338.1375) centre (-6.35, 341.3125) ccw
  line L3 (-6.35, 338.1375) -> (-3.175, 338.1375)
  arc A9 (-3.175, 338.1375) -> (0, 341.3125) centre (-3.175, 341.3125) ccw
  line L4 (0, 341.3125) -> (0, 352.425)
  arc A10 (0, 355.6) -> (0, 352.425) centre (0, 354.0125) ccw
  line L5 (0, 355.6) -> (1.5875, 355.6)
  arc A11 (4.7625, 355.6) -> (1.5875, 355.6) centre (3.175, 355.6) ccw
  line L6 (4.7625, 355.6) -> (4.7625, 95.25)
  arc A12 (3.175, 93.6625) -> (4.7625, 95.25) centre (3.175, 95.25) ccw
  line L7 (3.175, 93.6625) -> (-6.35, 93.6625)
  arc A13 (-6.35, 93.6625) -> (-9.525, 90.4875) centre (-6.35, 90.4875) ccw
  line L8 (-9.525, 90.4875) -> (-9.525, 61.9125)
  arc A14 (-9.525, 61.9125) -> (-6.35, 58.7375) centre (-6.35, 61.9125) ccw
  line L9 (-6.35, 58.7375) -> (-3.175, 58.7375)
  arc A15 (-3.175, 58.7375) -> (0, 61.9125) centre (-3.175, 61.9125) ccw
  line L10 (0, 61.9125) -> (0, 73.025)
  arc A16 (0, 76.2) -> (0, 73.025) centre (0, 74.6125) ccw
  line L11 (0, 76.2) -> (1.5875, 76.2)
  arc A17 (4.7625, 76.2) -> (1.5875, 76.2) centre (3.175, 76.2) ccw
  line L12 (4.7625, 76.2) -> (4.7625, 0)
  line L13 (4.7625, 0) -> (495.2375, 0)
  line L14 (498.4125, 76.2) -> (500, 76.2)
  line L15 (500, 73.025) -> (500, 61.9125)
  arc A18 (500, 61.9125) -> (503.175, 58.7375) centre (503.175, 61.9125) ccw
  line L16 (503.175, 58.7375) -> (506.35, 58.7375)
  arc A19 (506.35, 58.7375) -> (509.525, 61.9125) centre (506.35, 61.9125) ccw
  line L17 (509.525, 61.9125) -> (509.525, 90.4875)
  arc A20 (509.525, 90.4875) -> (506.35, 93.6625) centre (506.35, 90.4875) ccw
  line L18 (506.35, 93.6625) -> (496.825, 93.6625)
  arc A21 (495.2375, 95.25) -> (496.825, 93.6625) centre (496.825, 95.25) ccw
  line L19 (495.2375, 95.25) -> (495.2375, 355.6)
  line L20 (498.4125, 355.6) -> (500, 355.6)
  line L21 (500, 352.425) -> (500, 341.3125)
  arc A22 (500, 341.3125) -> (503.175, 338.1375) centre (503.175, 341.3125) ccw
  line L22 (503.175, 338.1375) -> (506.35, 338.1375)
  arc A23 (506.35, 338.1375) -> (509.525, 341.3125) centre (506.35, 341.3125) ccw
  line L23 (509.525, 341.3125) -> (509.525, 369.8875)
  arc A24 (509.525, 369.8875) -> (506.35, 373.0625) centre (506.35, 369.8875) ccw
  line L24 (506.35, 373.0625) -> (496.825, 373.0625)
  arc A25 (495.2375, 374.65) -> (496.825, 373.0625) centre (496.825, 374.65) ccw
  line L25 (495.2375, 374.65) -> (495.2375, 472.8122)
  line L26 (495.2375, 472.8122) -> (4.7625, 472.8122)
  line L27 (495.2375, 0) -> (495.2375, 76.2)
sketch "Side" plane through (0, 0, 0) normal (-1, 0, 0) x (0, -1, 0)
  arc A0 (-9.525, 390.525) -> (-9.525, 393.7) centre (-9.525, 392.1125) ccw
  line L0 (-9.525, 393.7) -> (-11.1125, 393.7)
  arc A1 (-11.1125, 393.7) -> (-14.2875, 393.7) centre (-12.7, 393.7) ccw
  line L1 (-14.2875, 393.7) -> (-14.2875, 355.6)
  arc A2 (-14.2875, 355.6) -> (-11.1125, 355.6) centre (-12.7, 355.6) ccw
  line L2 (-11.1125, 355.6) -> (-9.525, 355.6)
  arc A3 (-9.525, 355.6) -> (-9.525, 358.775) centre (-9.525, 357.1875) ccw
  line L3 (-9.525, 358.775) -> (-9.525, 390.525)
  arc A4 (-9.525, 111.125) -> (-9.525, 114.3) centre (-9.525, 112.7125) ccw
  line L4 (-9.525, 114.3) -> (-11.1125, 114.3)
  arc A5 (-11.1125, 114.3) -> (-14.2875, 114.3) centre (-12.7, 114.3) ccw
  line L5 (-14.2875, 114.3) -> (-14.2875, 76.2)
  arc A6 (-14.2875, 76.2) -> (-11.1125, 76.2) centre (-12.7, 76.2) ccw
  line L6 (-11.1125, 76.2) -> (-9.525, 76.2)
  arc A7 (-9.525, 76.2) -> (-9.525, 79.375) centre (-9.525, 77.7875) ccw
  line L7 (-9.525, 79.375) -> (-9.525, 111.125)
  arc A8 (-88.1651, 501.8727) -> (-91.201, 502.8022) centre (-89.6831, 502.3374) ccw
  line L8 (-91.201, 502.8022) -> (-101.8267, 506.0552)
  arc A9 (-103.9332, 510.0206) -> (-101.8267, 506.0552) centre (-100.8973, 509.0911) ccw
  line L9 (-103.9332, 510.0206) -> (-103.4685, 511.5386)
  arc A10 (-99.5031, 513.645) -> (-103.4685, 511.5386) centre (-100.4326, 510.6091) ccw
  line L10 (-99.5031, 513.645) -> (-72.1799, 505.2799)
  arc A11 (-70.0735, 501.3146) -> (-72.1799, 505.2799) centre (-73.1094, 502.244) ccw
  line L11 (-70.0735, 501.3146) -> (-72.3971, 493.7248)
  arc A12 (-72.3971, 493.7248) -> (-71.3439, 491.7421) centre (-70.8791, 493.2601) ccw
  line L12 (-71.3439, 491.7421) -> (-1.1228, 470.2437)
  arc A13 (0, 468.7258) -> (-1.1228, 470.2437) centre (-1.5875, 468.7258) ccw
  line L13 (0, 468.7258) -> (0, 1.5875)
  arc A14 (-1.5875, 0) -> (0, 1.5875) centre (-1.5875, 1.5875) ccw
  line L14 (-1.5875, 0) -> (-327.025, 0)
  arc A15 (-336.55, 9.525) -> (-327.025, 0) centre (-327.025, 9.525) ccw
  line L15 (-336.55, 9.525) -> (-336.55, 570.7895)
  arc A16 (-334.4978, 572.3074) -> (-336.55, 570.7895) centre (-334.9625, 570.7895) ccw
  line L16 (-334.4978, 572.3074) -> (-246.9907, 545.5169)
  arc A17 (-246.9899, 545.5193) -> (-246.0605, 548.5552) centre (-246.5252, 547.0372) ccw
  line L17 (-246.9907, 545.5169) -> (-246.9899, 545.5193)
  arc A18 (-245.5965, 550.0707) -> (-248.6324, 551.0002) centre (-247.1145, 550.5355) ccw
  line L18 (-248.6324, 551.0002) -> (-259.2581, 554.2533)
  arc A19 (-261.3645, 558.2186) -> (-259.2581, 554.2533) centre (-258.3286, 557.2892) ccw
  line L19 (-261.3645, 558.2186) -> (-260.8998, 559.7366)
  arc A20 (-256.9345, 561.843) -> (-260.8998, 559.7366) centre (-257.8639, 558.8071) ccw
  line L20 (-256.9345, 561.843) -> (-229.6113, 553.478)
  arc A21 (-227.5048, 549.5126) -> (-229.6113, 553.478) centre (-230.5407, 550.4421) ccw
  line L21 (-227.5048, 549.5126) -> (-229.8285, 541.9229)
  arc A22 (-229.8285, 541.9229) -> (-228.7752, 539.9402) centre (-228.3105, 541.4581) ccw
  line L22 (-228.7752, 539.9402) -> (-89.5593, 497.3188)
  arc A23 (-89.5586, 497.3212) -> (-88.6291, 500.3571) centre (-89.0939, 498.8392) ccw
  line L23 (-89.5593, 497.3188) -> (-89.5586, 497.3212)
  line L24 (-246.0605, 548.5552) -> (-245.5965, 550.0707)
  line L25 (-88.6291, 500.3571) -> (-88.1651, 501.8727)
sketch "Top" plane through (0, -132.9268, 434.1848) normal (0, -0.292741, 0.956192) x (1, 0, 0)
  arc A0 (500, 369.6221) -> (500, 372.7971) centre (500, 371.2096) ccw
  line L0 (500, 395.8655) -> (500, 372.7971)
  line L1 (495.2375, 357.7655) -> (495.2375, 395.8655)
  line L2 (495.2375, 395.8655) -> (500, 395.8655)
  line L3 (500, 193.1214) -> (495.2375, 193.1214)
  line L4 (495.2375, 193.1214) -> (495.2375, 231.2214)
  line L5 (495.2375, 231.2214) -> (500, 231.2214)
  line L6 (500, 231.2214) -> (500, 193.1214)
  arc A1 (500, 487.3122) -> (498.4125, 488.8997) centre (498.4125, 487.3122) ccw
  line L7 (498.4125, 488.8997) -> (1.5875, 488.8997)
  arc A2 (1.5875, 488.8997) -> (0, 487.3122) centre (1.5875, 487.3122) ccw
  line L8 (0, 487.3122) -> (0, 481.4602)
  arc A3 (-3.7197, 472.4799) -> (0, 481.4602) centre (-12.7, 481.4602) ccw
  line L9 (-3.7197, 472.4799) -> (-15.3303, 460.8694)
  arc A4 (-15.3303, 460.8694) -> (-19.05, 451.8892) centre (-6.35, 451.8892) ccw
  line L10 (-19.05, 451.8892) -> (-19.05, 119.1136)
  arc A5 (-19.05, 119.1136) -> (-6.35, 106.4136) centre (-6.35, 119.1136) ccw
  line L11 (-6.35, 106.4136) -> (506.35, 106.4136)
  arc A6 (506.35, 106.4136) -> (519.05, 119.1136) centre (506.35, 119.1136) ccw
  line L12 (519.05, 119.1136) -> (519.05, 451.8892)
  arc A7 (519.05, 451.8892) -> (515.3303, 460.8694) centre (506.35, 451.8892) ccw
  line L13 (515.3303, 460.8694) -> (503.7197, 472.4799)
  arc A8 (500, 481.4602) -> (503.7197, 472.4799) centre (512.7, 481.4602) ccw
  line L14 (500, 481.4602) -> (500, 487.3122)
  line L15 (0, 372.7971) -> (0, 395.8655)
  line L16 (0, 395.8655) -> (4.7625, 395.8655)
  line L17 (4.7625, 395.8655) -> (4.7625, 357.7655)
  line L18 (0, 231.2214) -> (4.7625, 231.2214)
  line L19 (4.7625, 231.2214) -> (4.7625, 193.1214)
  line L20 (4.7625, 193.1214) -> (0, 193.1214)
  line L21 (0, 193.1214) -> (0, 231.2214)
  line L22 (500, 369.6221) -> (500, 357.7655)
  arc A9 (0, 372.7971) -> (0, 369.6221) centre (0, 371.2096) ccw
  line L23 (4.7625, 357.7655) -> (0, 357.7655)
  line L24 (0, 357.7655) -> (0, 369.6221)
  line L25 (500, 357.7655) -> (495.2375, 357.7655)
component "Left Side" placed x (1, 0, 0) y (0, 1, 0) z (0, 0, 1) at (0, 0, 0)
component "Right Side" placed x (1, 0, 0) y (0, 1, 0) z (0, 0, 1) at (0, 0, 0)
component "Front" placed x (1, 0, 0) y (0, 1, 0) z (0, 0, 1) at (0, 0, 0)
component "Top" placed x (1, 0, 0) y (0, 1, 0) z (0, 0, 1) at (0, 0, 0)
equation "d1 = 50 cm - 1 in"
equation "d8 = d15"
equation "d9 = ( 3 / 16 ) * 1 in"
equation "d14 = ( 3 / 16 ) * 1 in"
equation "d22 = ( 3 / 16 ) * 1 in"
equation "d23 = ( 0.875 / 2 ) * 1 in"
equation "d26 = d23"
equation "d37 = ( 3 / 16 ) * 1 in"
equation "d77 = ( 3 / 16 ) * 1 in"
equation "d94 = d93"
equation "d97 = d92"
equation "d152 = d140"
equation "d153 = 1.5 in - 0.125 in"
equation "d154 = d153 / 2"
equation "d155 = ( 3 / 16 ) * 1 in"
equation "d159 = d154"
equation "d160 = d153"
equation "d161 = d159"
equation "d162 = d155"
equation "d163 = d162"
equation "d165 = d152"
equation "d203 = 1.5 in - 0.125 in"
equation "d204 = d203 / 2"
equation "d206 = 1.5 in - 0.125 in"
equation "d207 = d203 / 2"
equation "d208 = ( 1 / 8 ) * 1 in"
equation "d209 = ( 1 / 16 ) * 1 in"
equation "d224 = ( 1 / 16 ) * 1 in"
equation "d225 = d218"
equation "d228 = ( 1 / 8 ) * 1 in"
equation "d229 = ( 1 / 8 ) * 1 in"
equation "d230 = ( 1 / 8 ) * 1 in"
equation "d231 = ( 1 / 8 ) * 1 in"
equation "d232 = ( 1 / 8 ) * 1 in"
equation "d234 = ( 1 / 16 ) * 1 in"
equation "d235 = ( 1 / 16 ) * 1 in"
equation "d236 = d235"
named bodies: "Front", "Left Panel", "Right Panel", "Left Panel (1)"
